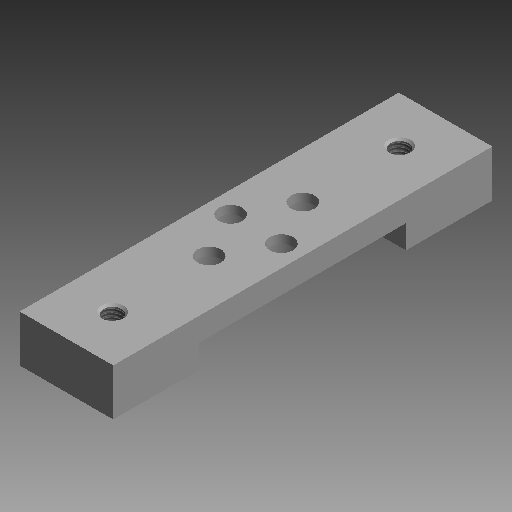
# Autodesk Inventor part: 25-2752-1_p
Saved by Autodesk Inventor 2019.4 (Build 234330000, 330)
## iProperties
Category: PARTsolutions
Company: 8020
Part Number: 25-2752-1_p
Material: Generic
Catalog Web Link: www.cadenas.de
Description: 25-2750, 25-2752, 40-2754, 40-2757, 25-2750-Black, 25-2752-Black, 40-2754-Black, 40-2757-Black_p-Roller Wheel Brackets
Vendor: 8020
Document SubType Name: Modeling
Designer: partserver
Manufacturer: 8020
Mass: 21.9882 g
Surface Area: 88.509 cm^2
Volume: 21.9882 cm^3
Density: 1 g/cm^3
Appearance: PSOLRGB-191-191-191
PSOL_IDENT_0: {$CADENAS_DATA\23d-libs\8020\metric\linear_motion\25_2750.prj},254 {VTYP=3D},{NB=25-2752-1_p},{LINA=
PSOL_IDENT_1: 25-2752-1_p},{NN=25-2750, 25-2752, 40-2754, 40-2757, 25-2750-Black, 25-2752-Black, 40-2754-Black, 40
PSOL_IDENT_2: -2757-Black_p},{DATE=31.07.2020 09:21:29},{GEOMDATE=19.09.2017 18:57:09},{VERSION=},{LINEID=20},{WBV
PSOL_IDENT_3: AR=MS},{WBNUMERIC=}  {NB=25-2752-1_p},{LINA=25-2752-1_p},{KT=DUMMY},{PN=25-2752},{MAT=Aluminum},{FIN=
PSOL_IDENT_4: Clear Anodize},{MS=1},{A=103.00},{B=78.00},{C=56.10},{D=64.20},{E=51.50},{F=25.40},{G=23.45},{H=12.5
PSOL_IDENT_5: 0},{J=6.40},{K=12.70},{L=25.40},{M=13.81},{N=12.70},{P=5.79},{Q=M6 x 1.00},{Q1=6.00000000},{R=M6},{R
PSOL_IDENT_6: 1=6.29920000},{RCB=10.31240000},{RCBD=4.01320000},{W=.064},{FT=0.08700000},{NO=1},{NO1=2},{CLR=.75,.
PSOL_IDENT_7: 75,.75}
NB: 25-2752-1_p
NN: 25-2750, 25-2752, 40-2754, 40-2757, 25-2750-Black, 25-2752-Black, 40-2754-Black, 40-2757-Black_p
NT: Roller Wheel Brackets
NBSYN: $PN.-$MS._p
LINA: 25-2752-1_p
CATALOG: 80/20
PN: 25-2752
MAT: Aluminum
FIN: Clear Anodize
A: 103
B: 78
C: 56.1
D: 64.2
E: 51.5
F: 25.4
G: 23.45
H: 12.5
J: 6.4
K: 12.7
L: 25.4
M: 13.81
N: 12.7
P: 5.79
Q: M6 x 1.00
Q1: 6
R: M6
R1: 6.2992
RCB: 10.3124
RCBD: 4.0132
W: .064
SUPPLIER: 8020
ARTICLENO: 25-2752-1_p
BOMINFO: 25-2752-1_p
CREATOR: CADENAS GmbH
Title: 25-2752-1_p
Author: Cadenas PARTsolutions
Comments: Roller Wheel Brackets
Autodesk Inventor part; units mm, degrees
ref_plane "YZ Plane" through (0, 0, 0) normal (1, 0, 0) x (0, 1, 0)
ref_plane "XZ Plane" through (0, 0, 0) normal (0, 1, 0) x (-1, 0, 0)
ref_plane "XY Plane" through (0, 0, 0) normal (0, 0, 1) x (1, 0, 0)
sketch "Sketch_1" plane through (0, 0, 0) normal (1, 0, 0) x (0, 1, 0)
  line L0 (-28.05, 6.4) -> (-51.5, 6.4)
  line L1 (-51.5, 6.4) -> (-51.5, -6.3)
  line L2 (-51.5, -6.3) -> (51.5, -6.3)
  line L3 (51.5, -6.3) -> (51.5, 6.4)
  line L4 (51.5, 6.4) -> (28.05, 6.4)
  line L5 (28.05, 6.4) -> (28.05, 0)
  line L6 (28.05, 0) -> (-28.05, 0)
  line L7 (-28.05, 0) -> (-28.05, 6.4)
  constraints: 16 end point
extrude "Extrusion1" add sketch "Sketch_1" along normal mid plane 25.4
sketch "Sketch_2" plane through (0, 0, 0) normal (1, 0, 0) x (0, 1, 0)
  line L0 (39, -6.3) -> (39, 6.4)
  line L1 (39, 6.4) -> (42, 6.4)
  line L2 (42, 6.4) -> (41.4585, 5.8585)
  line L3 (41.4585, 5.8585) -> (41.4585, -5.7585)
  line L4 (41.4585, -5.7585) -> (42, -6.3)
  line L5 (42, -6.3) -> (39, -6.3)
  line L6 (39, -6.3) -> (39, 6.4)
  constraints: 14 end point
revolve "Revolution1" cut sketch "Sketch_2" angle 360 about axis through (0, 39, -6.3) along (0, 0, -1)
thread "Thread1" size "M6x1" class "6H" standard "ISO Metric profile" full length
sketch "Sketch_3" plane through (0, 0, 0) normal (1, 0, 0) x (0, 1, 0)
  line L0 (-39, -6.3) -> (-39, 6.4)
  line L1 (-39, 6.4) -> (-36, 6.4)
  line L2 (-36, 6.4) -> (-36.5415, 5.8585)
  line L3 (-36.5415, 5.8585) -> (-36.5415, -5.7585)
  line L4 (-36.5415, -5.7585) -> (-36, -6.3)
  line L5 (-36, -6.3) -> (-39, -6.3)
  line L6 (-39, -6.3) -> (-39, 6.4)
  constraints: 14 end point
revolve "Revolution2" cut sketch "Sketch_3" angle 360 about axis through (0, -39, -6.3) along (0, 0, -1)
thread "Thread2" size "M6x1" class "6H" standard "ISO Metric profile" full length
sketch "Sketch4" plane through (-12.7, -28.05, 0) normal (0, 0, 1) x (1, 0, 0)
  point P0 (5.795, 28.05)
hole "Hole1" at (-6.905, 0, 0) direction (0, 0, -1) diameter 6.2992 depth 6.3 counterbore diameter 10.3124 counterbore depth 4.0132
pattern_linear "Rectangular Pattern1" count 2 spacing 14.4558 along (0.4776642, 0.8785425, 0) count 2 spacing 14.4558 along (0.4776642, -0.8785425, 0) of "Hole1"
ref_plane "screw1_XY" through (-6.905, 0, -4.0132) normal (0, 0, 1) x (1, 0, 0)
ref_plane "screw1_YZ" through (-6.905, 0, -4.0132) normal (1, 0, 0) x (0, 1, 0)
ref_plane "screw1_ZX" through (-6.905, 0, -4.0132) normal (0, 1, 0) x (0, 0, 1)
ref_plane "screw1_1_XY" through (0, 12.7, -4.0132) normal (0, 0, 1) x (1, 0, 0)
ref_plane "screw1_1_YZ" through (0, 12.7, -4.0132) normal (1, 0, 0) x (0, 1, 0)
ref_plane "screw1_1_ZX" through (0, 12.7, -4.0132) normal (0, 1, 0) x (0, 0, 1)
ref_plane "screw2_XY" through (6.905, 0, -4.0132) normal (0, 0, 1) x (1, 0, 0)
ref_plane "screw2_YZ" through (6.905, 0, -4.0132) normal (1, 0, 0) x (0, 1, 0)
ref_plane "screw2_ZX" through (6.905, 0, -4.0132) normal (0, 1, 0) x (0, 0, 1)
ref_plane "screw2_1_XY" through (0, -12.7, -4.0132) normal (0, 0, 1) x (1, 0, 0)
ref_plane "screw2_1_YZ" through (0, -12.7, -4.0132) normal (1, 0, 0) x (0, 1, 0)
ref_plane "screw2_1_ZX" through (0, -12.7, -4.0132) normal (0, 1, 0) x (0, 0, 1)
ref_plane "to_dummy_XY" through (0, 0, 0) normal (0, 0, 1) x (1, 0, 0)
ref_plane "to_dummy_YZ" through (0, 0, 0) normal (1, 0, 0) x (0, 1, 0)
ref_plane "to_dummy_ZX" through (0, 0, 0) normal (0, 1, 0) x (0, 0, 1)
ref_plane "to_wheel1_XY" through (0, 39, 6.4) normal (0, 0, 1) x (1, 0, 0)
ref_plane "to_wheel1_YZ" through (0, 39, 6.4) normal (1, 0, 0) x (0, 1, 0)
ref_plane "to_wheel1_ZX" through (0, 39, 6.4) normal (0, 1, 0) x (0, 0, 1)
ref_plane "to_wheel2_XY" through (0, -39, 6.4) normal (0, 0, 1) x (1, 0, 0)
ref_plane "to_wheel2_YZ" through (0, -39, 6.4) normal (1, 0, 0) x (0, 1, 0)
ref_plane "to_wheel2_ZX" through (0, -39, 6.4) normal (0, 1, 0) x (0, 0, 1)
body "Solid1"
